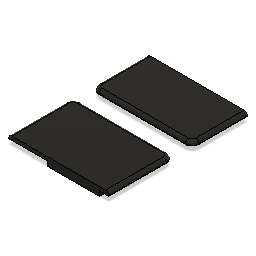
Afdekplaatje v5 (Autodesk Fusion 360 design; units mm, degrees)
Autodesk Fusion 360 part; units mm, degrees
sketch "Sketch1" plane through (0, 0, 0) normal (0, 1, 0) x (1, 0, 0)
  line L0 (-55, -64) -> (0, -64)
  line L1 (0, 0) -> (-81, 0)
  line L2 (-81, 0) -> (-81, -44)
  line L3 (-55, -44) -> (-55, -64)
  line L4 (-81, -44) -> (-55, -44)
  line L5 (0, -64) -> (0, 0)
  line L6 (-55, 84) -> (0, 84)
  line L7 (-87, 30) -> (-87, 75)
  line L8 (0, 30) -> (-87, 30)
  line L9 (-55, 84) -> (-55, 75)
  line L10 (0, 84) -> (0, 30)
  line L11 (-55, 75) -> (-87, 75)
  line L12 (-97, 84) -> (10, 84)
  line L13 (10, 84) -> (10, 25)
  line L14 (10, 25) -> (-97, 25)
  line L15 (-97, 25) -> (-97, 84)
  line L16 (-97, 5) -> (10, 5)
  line L17 (10, 5) -> (10, -64)
  line L18 (10, -64) -> (-97, -64)
  line L19 (-97, -64) -> (-97, 5)
  dimension "d2" = 26
  dimension "d4" = 81
  dimension "d5" = 64
  dimension "d6" = 20
  dimension "d9" = 9
  dimension "d10" = 32
  dimension "d11" = 54
  dimension "d12" = 87
  dimension "d13" = 10
  dimension "d15" = 5
  dimension "d16" = 10
  dimension "d17" = 5
  dimension "d18" = 10
  constraint horizontal L0
  constraint vertical L5
  constraint horizontal L1
  constraint vertical L2
  constraint perpendicular L2 L4
  constraint perpendicular L0 L3
  constraint coincident L1.start L5.end
  constraint horizontal L6
  constraint vertical L10
  constraint horizontal L8
  constraint vertical L7
  constraint perpendicular L7 L11
  constraint perpendicular L9 L11
  constraint horizontal L12
  constraint vertical L13
  constraint horizontal L14
  constraint vertical L15
  constraint collinear L6 L12
  constraint horizontal L16
  constraint vertical L17
  constraint horizontal L18
  constraint vertical L19
  constraint collinear L0 L18
  constraint collinear L13 L17
  constraint collinear L15 L19
  measures "d2" distance of L2.end L3.start
  measures "d4" distance of L1.start L1.end
  measures "d5" distance of L1.start L0.end
  measures "d6" distance of L3.start L0.start
  measures "d9" distance of L6.start L9.end
  measures "d10" distance of L9.end L7.end
  measures "d11" distance of L6.end L8.start
  measures "d12" distance of L8.start L7.start
  measures "d13" distance of L10 L13
  measures "d15" distance of L8 L14
  measures "d16" distance of L5 L17
  measures "d17" distance of L1 L16
  measures "d18" distance of L7 L15
extrude "Extrude1" add sketch "Sketch1" along normal blind 5 contours L0 L1 L2 L3 L4 L5 L18 | L6 L7 L8 L9 L10 L11 L12 makes body 1 at (-18.3333, 0, 36) makes body 2 at (-47.3333, 0, -45)
extrude "Extrude2" add sketch "Sketch1" along normal blind 4 from surface at 5 bodies 1 2
fillet "Fillet1" radius 7.5 4 edges at (10, 7, -5) (-97, 7, -5) (-97, 7, -25) (10, 7, -25) on bodies 1 2
fillet "Fillet2" radius 3.5 10 edges at (10, 9, 33.25) (7.8033, 9, -2.8033) (-43.5, 9, -5) (-94.8033, 9, -2.8033) (-97, 9, 33.25) (-97, 9, -58.25) (-94.8033, 9, -27.1967) (-43.5, 9, -25) (7.8033, 9, -27.1967) (10, 9, -58.25) on bodies 1 2
copy_body "Body->Comp1" bodies 2 removing the originals makes body 3 in component "Component"
copy_body "Body->Comp2" bodies 1 removing the originals makes body 4 in component "Component'"
component "Component" placed x (1, 0, 0) y (0, 1, 0) z (0, 0, 1) at (0, 0, 0)
component "Component'" placed x (1, 0, 0) y (0, 1, 0) z (0, 0, 1) at (0, 0, 0)
